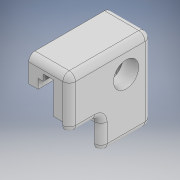
# Autodesk Inventor part: Rubber_Gromment_Cap_LM6015
Saved by Autodesk Inventor 2020.3 (Build 243373000, 373)
## iProperties
Created: 2020-04-20
Part Number: Rubber_Gromment_Cap_LM6015
Material: Generic
Document SubType Name: Modeling
Designer: rah75
Density: 1 g/cm^3
Appearance: Default
Author: rah75
Autodesk Inventor part; units mm, degrees
ref_plane "YZ Plane" through (0, 0, 0) normal (1, 0, 0) x (0, 1, 0)
ref_plane "XZ Plane" through (0, 0, 0) normal (0, 1, 0) x (-1, 0, 0)
ref_plane "XY Plane" through (0, 0, 0) normal (0, 0, 1) x (1, 0, 0)
sketch "Sketch1" plane through (0, 0, 0) normal (0, 0, 1) x (1, 0, 0)
  line L0 (-2, 2) -> (-2, 7)
  line L1 (-2, 7) -> (-3, 7)
  line L2 (-3, 7) -> (-3, 8)
  line L3 (-3, 8) -> (0, 8)
  line L4 (0, 8) -> (0, 2)
  line L5 (0, 2) -> (-2, 2)
  line L6 (0, 0) -> (-1.3687, 0) construction
  dimension "d0" = 14
  dimension "d1" = 1
  dimension "d2" = 1
  dimension "d3" = 2
  dimension "d4" = 4
  constraints: 14 end point, 5 perpendicular, 1 horizontal, 1 point on line, 1 vertical
  measures "d0" diameter of L1 L6
  measures "d1" distance of L0.end L1.end
  measures "d2" distance of L1.end L2.end
  measures "d3" distance of L4.end L0.start
  measures "d4" diameter of L5 L6
revolve "Revolution1" add sketch "Sketch1" angle 360 about axis through (0, 0, 0) along (-1, 0, 0)
sketch "Sketch2" plane through (0, 0, 0) normal (1, 0, 0) x (0, 0, -1)
  line L0 (3, 3) -> (-8, 3)
  line L1 (-8, 3) -> (-8, -8)
  line L2 (-8, -8) -> (3, -8)
  line L3 (3, -8) -> (3, 3)
  circle A0 centre (0, 0) radius 8 projected
  point P0 (-7.4162, 3)
  point P1 (3, -7.4162)
  dimension "d6" = 3
  dimension "d7" = 3
  constraints: 8 end point, 2 parallel, 2 tangent, 1 horizontal, 1 perpendicular
  measures "d6" distance from line of point (0, 0) L3
  measures "d7" distance from line of L0 point (0, 0)
extrude "Extrusion1" add sketch "Sketch2" along normal blind 1.651 contours L0 A0 L3 picked at (3.5531, -3.6398)
sketch "Sketch3" plane through (-3, 0, 0) normal (-1, 0, 0) x (0, 0, 1)
  circle A0 centre (0, 0) radius 7 projected
  circle A1 centre (0, 0) radius 8 projected
  line L0 (8, -8) -> (-8, -8)
  line L1 (-8, -8) -> (-8, 8)
  line L2 (-8, 8) -> (8, 8)
  line L3 (8, 8) -> (8, -8)
  line L4 (8, -8) -> (-8, 8) construction
  line L5 (-8, -8) -> (8, 8) construction
  point P0 (8, 0)
  point P1 (0, 8)
  point P2 (-8, 0)
  point P3 (0, -8)
  constraints: 12 end point, 2 midpoint, 2 parallel, 2 tangent, 1 horizontal, 1 perpendicular
extrude "Extrusion2" add sketch "Sketch3" against normal up to surface (4.651 mm away) contours A1 L2 L3 | A1 L1 L2 | L0 L1 A1
sketch "Sketch4" plane through (0, -7.4162, -3) normal (1, 0, 0) x (0, 0, -1)
  line L0 (0, 10.4162) -> (-10.4162, 10.4162) projected
  line L1 (0, 10.4162) -> (-13.5141, 10.4162)
  line L2 (-13.5141, 10.4162) -> (-13.5141, -2.0306)
  line L3 (-13.5141, -2.0306) -> (0, -2.0306)
  line L4 (0, -2.0306) -> (0, 10.4162)
  point P0 (-3, 7.4162)
  constraints: 8 end point, 2 parallel, 1 horizontal, 1 perpendicular
extrude "Extrusion3" cut sketch "Sketch4" along normal blind 10
sketch "Sketch5" plane through (1.651, 0, 0) normal (1, 0, 0) x (0, 0, -1)
  line L0 (3, 3) -> (3, -8) projected
  line L1 (8, -8) -> (3, -8) projected
  line L2 (8, 8) -> (8, -8) projected
  line L3 (-8, 8) -> (8, 8) projected
  line L4 (-8, 3) -> (-8, 8) projected
  line L5 (-8, 3) -> (3, 3) projected
  line L6 (-8, -8) -> (5, -8)
  line L7 (5, -8) -> (5, 5)
  line L8 (5, 5) -> (-8, 5)
  line L9 (-8, 5) -> (-8, -8)
  line L10 (-8, -8) -> (5, 5) construction
  line L11 (5, -8) -> (-8, 5) construction
  circle A0 centre (0, 0) radius 2 projected
  point P0 (-1.5, -1.5)
  dimension "d16" = 5
  dimension "d17" = 5
  constraints: 12 end point, 2 collinear, 2 midpoint, 2 parallel, 1 horizontal, 1 perpendicular
  measures "d16" distance from line of A0.centre L7
  measures "d17" distance from line of A0.centre L8
extrude "Extrusion4" add sketch "Sketch5" along normal blind 3.175 contours L7 L8 L4 L3 L2 L1
sketch "Sketch6" plane through (4.826, 0, 0) normal (1, 0, 0) x (0, 0, -1)
  line L0 (-8, -8) -> (8, -8)
  line L1 (8, -8) -> (8, 8)
  line L2 (8, 8) -> (-8, 8)
  line L3 (-8, 8) -> (-8, -8)
  line L4 (-8, -8) -> (8, 8) construction
  line L5 (8, -8) -> (-8, 8) construction
  line L6 (8, -8) -> (8, 8) projected
  line L7 (8, 8) -> (-8, 8) projected
  circle A0 centre (0, 0) radius 4
  line L8 (5, 5) -> (5, -8) projected
  line L9 (-8, 5) -> (5, 5) projected
  point P0 (0, 0)
  dimension "d20" = 8
  constraints: 12 end point, 2 collinear, 2 midpoint, 2 parallel, 2 point on line, 1 centre point, 1 coincident, 1 horizontal, 1 perpendicular
  measures "d20" diameter of A0
extrude "Extrusion5" add sketch "Sketch6" along normal blind 5
sketch "Sketch7" plane through (4.826, 0, 0) normal (-1, 0, 0) x (0, 0, 1)
  line L0 (8, -8) -> (5, -8)
  line L1 (5, -8) -> (5, -5)
  line L2 (5, -5) -> (8, -5)
  line L3 (8, -5) -> (8, -8)
  line L4 (8, -8) -> (5, -5) construction
  line L5 (5, -8) -> (8, -5) construction
  line L6 (-5, 5) -> (-5, -8) projected
  line L7 (8, 5) -> (-5, 5) projected
  point P0 (0, 0)
  point P1 (6.5, -6.5)
  dimension "d26" = 10
  dimension "d27" = 10
  constraints: 12 end point, 2 midpoint, 2 parallel, 1 coincident, 1 horizontal, 1 perpendicular
  measures "d26" distance between parallel lines of L1 L6
  measures "d27" distance between parallel lines of L7 L2
extrude "Extrusion6" cut sketch "Sketch7" against normal blind 3
sketch "Sketch8" plane through (-3, -8, -8) normal (0, -1, 0) x (1, 0, 0)
  line L0 (10.826, 16) -> (10.826, 13) projected
  line L1 (10.826, 13) -> (7.826, 13) projected
  line L2 (7.826, 13) -> (7.826, 3) projected
  line L3 (4.651, 3) -> (7.826, 3) projected
  line L4 (4.651, 3) -> (4.651, 5) projected
  line L5 (4.651, 5) -> (3, 5) projected
  line L6 (3, 5) -> (3, 8) projected
  line L7 (0, 8) -> (3, 8) projected
  line L8 (0, 0) -> (0, 8) projected
  line L9 (0, 0) -> (12.826, 0) projected
  line L10 (12.826, 16) -> (12.826, 0) projected
  line L11 (10.826, 16) -> (12.826, 16) projected
  point P0 (3, 8)
extrude "Extrusion7" add sketch "Sketch8" along normal blind 10
sketch "Sketch9" plane through (-3, 0, 8) normal (0, 0, 1) x (1, 0, 0)
  line L0 (10.826, -5) -> (10.826, -18) projected
  line L1 (12.826, -18) -> (10.826, -18) projected
  line L2 (12.826, 8) -> (12.826, -18) projected
  line L3 (0, 8) -> (12.826, 8) projected
  line L4 (0, 0) -> (0, 8) projected
  line L5 (0, 0) -> (3, 0) projected
  line L6 (3, 0) -> (3, 3) projected
  line L7 (3, 3) -> (4.651, 3) projected
  line L8 (4.651, 3) -> (4.651, 5) projected
  line L9 (4.651, 5) -> (7.826, 5) projected
  line L10 (7.826, 5) -> (7.826, -5) projected
  line L11 (7.826, -5) -> (10.826, -5) projected
  point P0 (3, 0)
extrude "Extrusion8" add sketch "Sketch9" along normal blind 10
sketch "Sketch10" plane through (7.826, 0, 0) normal (-1, 0, 0) x (0, 0, 1)
  line L0 (5, -5) -> (18, -5) projected
  line L1 (5, -18) -> (5, -5) projected
  line L2 (5, -18) -> (18, -18) projected
  line L3 (18, -5) -> (18, -18) projected
  line L4 (8, -8) -> (18, -8)
  line L5 (18, -8) -> (18, -18)
  line L6 (18, -18) -> (8, -18)
  line L7 (8, -18) -> (8, -8)
  line L8 (8, -8) -> (18, -18) construction
  line L9 (18, -8) -> (8, -18) construction
  point P0 (0, 0)
  point P1 (13, -13)
  point P2 (8, -18)
  dimension "d34" = 3
  dimension "d35" = 3
  constraints: 12 end point, 2 midpoint, 2 parallel, 1 horizontal, 1 perpendicular
  measures "d34" distance between parallel lines of L1 L7
  measures "d35" distance between parallel lines of L0 L4
extrude "Extrusion9" cut sketch "Sketch10" against normal blind 10 contours L3 L2 L7 L4
fillet "Fillet1" radius 2 2 edges at (-1.5, -8, 0) (-1.5, 0, 8)
fillet "Fillet2" radius 2 6 edges at (8.826, -8, 18) (8.826, -18, 8) (8.826, -8, 8) (3.413, 8, -8) (3.413, -18, -8) (3.413, 8, 18)
fillet "Fillet3" radius 2 12 edges at (9.826, 7.4142, 17.4142) (9.826, 0, 18) (9.826, -7.4142, 17.4142) (9.826, -8, 13) (9.826, -8.5858, 8.5858) (9.826, -13, 8) (9.826, -17.4142, 7.4142) (9.826, -18, 0) (9.826, -17.4142, -7.4142) (9.826, -5, -8) (9.826, 7.4142, -7.4142) (9.826, 8, 5)
equation "\"d7\" = d6"
equation "\"d27\" = d26"
body "Solid1"
